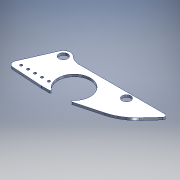
# Autodesk Inventor part: Flywheel Bracket 1
Saved by Autodesk Inventor 2019.4 (Build 234330000, 330)
## iProperties
Created: 2020-01-06
Part Number: Flywheel Bracket 1
Material: Aluminum 6061
Document SubType Name: Modeling
Designer: admin
Density: 2.7 g/cm^3
Appearance: Aluminum - Flat
Author: admin
Autodesk Inventor part; units mm, degrees
ref_plane "YZ Plane" through (0, 0, 0) normal (1, 0, 0) x (0, 1, 0)
ref_plane "XZ Plane" through (0, 0, 0) normal (0, 1, 0) x (-1, 0, 0)
ref_plane "XY Plane" through (0, 0, 0) normal (0, 0, 1) x (1, 0, 0)
sketch "Sketch1" plane through (0, 0, 0) normal (0, 1, 0) x (-1, 0, 0)
  circle A0 centre (0, 0) radius 9.5
  circle A1 centre (77.0362, 35.9226) radius 9.5 construction
  line L0 (77.0362, 35.9226) -> (0, 0) construction
  line L1 (144.189, -12) -> (-82.3554, -12)
  line L2 (-82.3554, -12) -> (-31.0868, 43.4655)
  line L3 (-31.0868, 43.4655) -> (62.6574, 68.4226)
  line L4 (62.6574, 68.4226) -> (64.0458, 68.4226)
  arc A2 (109.5362, 35.9226) -> (85.4876, 4.5407) centre (77.0362, 35.9226) ccw construction
  circle A3 centre (0, 0) radius 40
  circle A4 centre (156.3912, 1.314) radius 9.5
  circle A5 centre (156.3912, 1.314) radius 15
  arc A6 (152.3238, -13.124) -> (144.189, -12) centre (144.189, -42) ccw
  line L5 (170.1336, -4.6982) -> (205.1336, 75.3018)
  line L6 (205.1336, 75.3018) -> (125.1336, 68.4226)
  arc A7 (64.0458, 68.4226) -> (90.0265, 68.4226) centre (77.0362, 35.9226) ccw
  line L7 (90.0265, 68.4226) -> (125.1336, 68.4226)
  line L8 (64.0458, 68.4226) -> (90.0265, 68.4226) construction
  arc A8 (90.0265, 68.4226) -> (64.0458, 68.4226) centre (77.0362, 35.9226) ccw construction
  dimension "d0" = 19
  dimension "d1" = 19
  dimension "d2" = 85
  dimension "d3" = 65
  dimension "d4" = 80
  dimension "d5" = 12
  dimension "d6" = 50
  dimension "d7" = 25
  dimension "d12" = 19
  dimension "d13" = 30
  dimension "d14" = 30
  dimension "d16" = 70
  dimension "d18" = 35
  dimension "d19" = 80
  dimension "d20" = 80
  constraints: 18 end point, 10 point on circle, 9 centre point, 6 coincident, 6 tangent, 3 parallel, 1 horizontal, 1 other
  measures "d0" diameter of A0
  measures "d1" diameter of A1
  measures "d2" distance of L0.start L0.end
  measures "d3" diameter of A2
  measures "d4" diameter of A3
  measures "d5" distance from line of L0.end L1
  measures "d6" distance from line of A3.centre L3
  measures "d7" angle of L1 L0
  measures "d12" diameter of A4
  measures "d13" diameter of A5
  measures "d14" radius of A6
  measures "d16" diameter of A7
  measures "d18" horizontal distance of L5.start L5.end
  measures "d19" vertical distance of L5.start L5.end
  measures "d20" horizontal distance of L5.end L6.end
extrude "Extrusion1" add sketch "Sketch1" along normal blind 5 contours L1 A3 L2 L3 L4 A7 L7 L6 L5 A5 A6 | L1 A3 | A5 picked at (-13.2582, 26.5327)
fillet "Fillet1" radius 5 1 edges at (82.3554, 2.5, -12)
fillet "Fillet2" radius 100 3 edges at (31.0868, 2.5, 43.4655) (-62.6574, 2.5, 68.4226) (-144.189, 2.5, -12)
fillet "Fillet3" radius 10 2 edges at (-205.1336, 2.5, 75.3018) (-125.1336, 2.5, 68.4226)
fillet "Fillet4" radius 2 2 edges at (-90.0265, 2.5, 68.4226) (-64.0458, 2.5, 68.4226)
sketch "Sketch2" plane through (0, 5, 0) normal (0, 1, 0) x (1, 0, 0)
  circle A0 centre (-178.1295, -61.3972) radius 2.75 projected
  circle A1 centre (-163.1295, -61.3972) radius 2.75 projected
  circle A2 centre (-148.1295, -61.3972) radius 2.75 projected
  circle A3 centre (-133.1295, -61.3972) radius 2.75 projected
  circle A4 centre (-118.1295, -61.3972) radius 2.75 projected
  point P0 (0, 0)
extrude "Extrusion2" cut sketch "Sketch2" against normal through all
body "Solid1"
